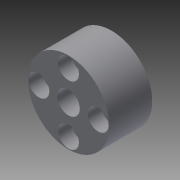
# Autodesk Inventor part: adaptor
Saved by Autodesk Inventor 2015 (Build 190159000, 159)
## iProperties
Created: 2014-10-25
Part Number: adaptor
Material: Generic
Document SubType Name: Modeling
Designer: jesse
Density: 1 g/cm^3
Appearance: Default
Author: jesse
Autodesk Inventor part; units mm, degrees
ref_plane "YZ Plane" through (0, 0, 0) normal (1, 0, 0) x (0, 1, 0)
ref_plane "XZ Plane" through (0, 0, 0) normal (0, 1, 0) x (-1, 0, 0)
ref_plane "XY Plane" through (0, 0, 0) normal (0, 0, 1) x (1, 0, 0)
sketch "Sketch1" plane through (0, 0, 0) normal (0, 0, 1) x (1, 0, 0)
  circle A0 centre (0, 0) radius 11
  circle A1 centre (0, 0) radius 3.05
  circle A2 centre (-8, 0) radius 1.3525
  circle A3 centre (0, 8) radius 1.3525
  circle A4 centre (8, 0) radius 1.3525
  circle A5 centre (0, -8) radius 1.3525
  constraints: 6 centre point
extrude "Extrusion1" add sketch "Sketch1" along normal blind 7.9375
sketch "Sketch6" plane through (0, 0, 7.9375) normal (0, 0, 1) x (1, 0, 0)
  circle A0 centre (0, 0) radius 3.05 projected
  circle A1 centre (0, -8) radius 1.3525 construction
  circle A2 centre (8, 0) radius 1.3525 construction
  circle A3 centre (0, 8) radius 1.3525 construction
  circle A4 centre (-8, 0) radius 1.3525 construction
  circle A5 centre (0, 0) radius 11 projected
  circle A6 centre (0, -8) radius 1.3525 projected
  circle A7 centre (0, -8) radius 2.8194
  circle A8 centre (8, 0) radius 2.8194
  circle A9 centre (0, 8) radius 2.8194
  circle A10 centre (-8, 0) radius 2.8194
  dimension "d12" = 5.6388
  constraints: 4 centre point, 4 coincident, 3 equal radius
  measures "d12" diameter of A7
extrude "Extrusion6" add sketch "Sketch6" along normal blind 3.683 contours A5
body "Solid1"
